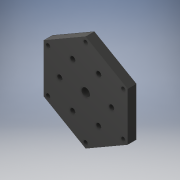
# Autodesk Inventor part: TA01
Saved by Autodesk Inventor 2017 (Build 210142000, 142)
## iProperties
Created: 2018-10-09
Part Number: TA01
Material: ABS Plastic
Document SubType Name: Modeling
Designer: Zach
Density: 1.06 g/cm^3
Appearance: Smooth - Black
Author: Zach
Autodesk Inventor part; units mm, degrees
ref_plane "YZ Plane" through (0, 0, 0) normal (1, 0, 0) x (0, 1, 0)
ref_plane "XZ Plane" through (0, 0, 0) normal (0, 1, 0) x (-1, 0, 0)
ref_plane "XY Plane" through (0, 0, 0) normal (0, 0, 1) x (1, 0, 0)
sketch "Sketch1" plane through (0, 0, 0) normal (0, 0, 1) x (1, 0, 0)
  circle A0 centre (0, 0) radius 5
  circle A1 centre (-30, 0) radius 3
  circle A2 centre (-15, -25.9808) radius 3
  circle A3 centre (15, -25.9808) radius 3
  circle A4 centre (30, 0) radius 3
  circle A5 centre (15, 25.9808) radius 3
  circle A6 centre (-15, 25.9808) radius 3
  line L0 (0, 56) -> (48.4974, 28)
  line L1 (48.4974, 28) -> (48.4974, -28)
  line L2 (48.4974, -28) -> (0, -56)
  line L3 (0, -56) -> (-48.4974, -28)
  line L4 (-48.4974, -28) -> (-48.4974, 28)
  line L5 (-48.4974, 28) -> (0, 56)
  point P0 (48.4974, 0)
  dimension "d0" = 10
  dimension "d2" = 6
  dimension "d6" = 360
  dimension "d15" = 30
  dimension "d33" = 112
  constraints: 12 end point, 7 centre point, 2 coincident, 2 horizontal alignment, 1 midpoint, 26 other
  measures "d0" diameter of A0
  measures "d2" diameter of A1
  measures "d15" distance of point (0, 0) A1.centre
  measures "d33" distance of L2.end L0.start
extrude "Extrusion1" add sketch "Sketch1" along normal blind 10
sketch "Sketch6" plane through (0, 0, 10) normal (0, 0, 1) x (1, 0, 0)
  circle A0 centre (0, 0) radius 5 construction
  circle A1 centre (-15, 25.9808) radius 3 construction
  circle A2 centre (15, 25.9808) radius 3 construction
  circle A3 centre (30, 0) radius 3 construction
  circle A4 centre (15, -25.9808) radius 3 construction
  circle A5 centre (-15, -25.9808) radius 3 construction
  circle A6 centre (-30, 0) radius 3 construction
  line L0 (48.4974, 28) -> (0, 56) construction
  line L1 (0, 56) -> (-48.4974, 28) construction
  line L2 (-48.4974, 28) -> (-48.4974, -28) construction
  line L3 (-48.4974, -28) -> (0, -56) construction
  line L4 (0, -56) -> (48.4974, -28) construction
  line L5 (48.4974, -28) -> (48.4974, 28) construction
  line L6 (-43.4974, 25.1132) -> (0, 50.2265)
  line L7 (0, 50.2265) -> (43.4974, 25.1132)
  line L8 (43.4974, 25.1132) -> (43.4974, -25.1132)
  line L9 (43.4974, -25.1132) -> (0, -50.2265)
  line L10 (0, -50.2265) -> (-43.4974, -25.1132)
  line L11 (-43.4974, -25.1132) -> (-43.4974, 25.1132)
  circle A7 centre (0, 50.2265) radius 2.5
  circle A8 centre (-43.4974, 25.1132) radius 2.5
  circle A9 centre (-43.4974, -25.1132) radius 2.5
  circle A10 centre (0, -50.2265) radius 2.5
  circle A11 centre (43.4974, -25.1132) radius 2.5
  circle A12 centre (43.4974, 25.1132) radius 2.5
  dimension "d34" = 5
  dimension "d35" = 5
  dimension "d38" = 360
  constraints: 12 end point, 6 centre point, 1 coincident, 18 other
  measures "d34" distance between parallel lines of L1 L6
  measures "d35" diameter of A7
extrude "Extrusion5" cut sketch "Sketch6" against normal through all contours L11 A8 L6 | L6 A8 L11 | A7 L7 L6 | L6 L7 A7 | A9 L10 L11 | L11 L10 A9 | A12 L8 L7 | L7 L8 A12 | A10 L9 L10 | L10 L9 A10 | A11 L9 L8 | L8 L9 A11
body "Solid1"
